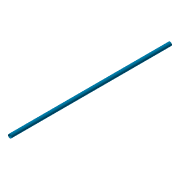
# Autodesk Inventor part: sparHoriz_B
Saved by Autodesk Inventor 2016 (Build 200138000, 138)
## iProperties
Company: HERA Project
Created: 2013-06-07
Part Number: sparHoriz_B
Material: PVC-Piping
Document SubType Name: Modeling
Designer: David DeBoer
Density: 1.4 g/cm^3
Description: Hub radial support spar
Mass: 1725.45 g
Surface Area: 6317.01 cm^2
Volume: 1232.47 cm^3
Appearance: Smooth - White
Author: David DeBoer
Title: Hub support spar
Autodesk Inventor part; units mm, degrees
ref_plane "YZ Plane" through (0, 0, 0) normal (1, 0, 0) x (0, 1, 0)
sketch "Sketch1" plane through (0, 0, 0) normal (0, 0, 1) x (1, 0, 0)
  circle A0 centre (0, 0) radius 31.5
  circle A1 centre (0, 0) radius 27.9
  dimension "d0" = 63
  dimension "d2" = 3.6
  constraints: 2 centre point, 1 coincident
  measures "d0" diameter of A0
  measures "d2" radial gap between concentric circles of A1 A0
extrude "Extrusion1" add sketch "Sketch1" along normal blind 2720
sketch "Sketch4" plane through (0, 0, 2720) normal (0, 0, 1) x (1, 0, 0)
  circle A0 centre (0, 0) radius 27.9 projected
  circle A1 centre (0, 0) radius 31.5 projected
  point P0 (0, 31.5)
  constraints: 1 vertical alignment, 1 other
ref_plane "Work Plane2" through (0, 31.5, 2720) normal (0, 1, 0) x (-1, 0, 0)
sketch "Sketch5" plane through (0, 31.5, 2720) normal (0, 1, 0) x (-1, 0, 0)
  circle A0 centre (0, -20) radius 2.0895
  line L0 (31.5, 0) -> (-31.5, 0) projected
  point P0 (0, -2720)
  dimension "d16" = 20
  constraints: 1 centre point
  measures "d16" distance from line of A0.centre L0
hole "Hole2" at (0, 31.5, 2700) direction (0, -1, 0) diameter 4.5 end through all
ref_plane "Work Plane3" through (0, 30, 0) normal (0, 1, 0) x (-1, 0, 0)
sketch "Sketch6" plane through (0, 30, 0) normal (0, 1, 0) x (-1, 0, 0)
  line L0 (-12.0739, 2711.7079) -> (13.0933, 2711.7079)
  line L1 (13.0933, 2711.7079) -> (13.0933, 2720)
  line L2 (13.0933, 2720) -> (-12.0739, 2720)
  line L3 (-12.0739, 2720) -> (-12.0739, 2711.7079)
  line L4 (31.5, 2720) -> (-31.5, 2720) projected
  point P0 (0, 0)
  dimension "d28" = 0
  dimension "d29" = 8.2921
  constraints: 8 end point, 2 parallel, 1 horizontal, 1 perpendicular
  measures "d28" distance between parallel lines of L4 L2
  measures "d29" distance of L2.end L0.start
extrude "Extrusion2" [suppressed]
body "Solid1"
